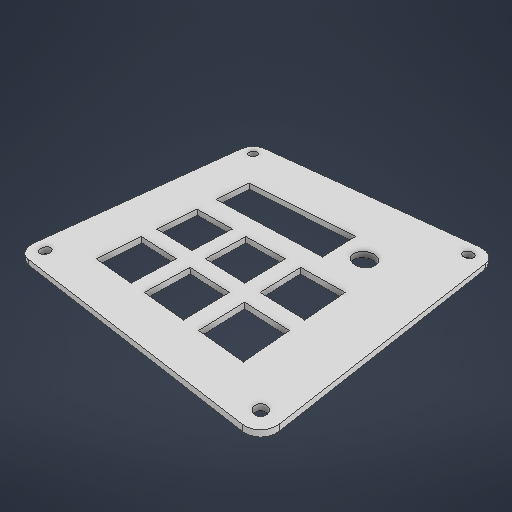
# Autodesk Inventor part: Case_Top
Saved by Autodesk Inventor 2026.1 (Build 301233000, 233)
## iProperties
Created: 2025-12-06
Part Number: Case_Top
Material: Generic
Document SubType Name: Modeling
Designer: chest
Density: 1 g/cm^3
Appearance: Default
Author: chest
Autodesk Inventor part; units mm, degrees
ref_plane "YZ Plane" through (0, 0, 0) normal (1, 0, 0) x (0, 1, 0)
ref_plane "XZ Plane" through (0, 0, 0) normal (0, 1, 0) x (-1, 0, 0)
ref_plane "XY Plane" through (0, 0, 0) normal (0, 0, 1) x (1, 0, 0)
sketch "Sketch1" plane through (0, 0, 0) normal (0, 1, 0) x (-1, 0, 0)
  line L0 (10.136, 16.6006) -> (-75.904, 16.6006)
  line L1 (-75.904, 16.6006) -> (-75.904, -66.8994)
  line L2 (-75.904, -66.8994) -> (10.136, -66.8994)
  line L3 (10.136, -66.8994) -> (10.136, 16.6006)
  point P0 (0, 0)
  dimension "d0" = 86.04
  dimension "d1" = 83.5
  constraints: 8 end point, 2 parallel, 1 horizontal, 1 perpendicular
  measures "d0" distance of L2.end L1.end
  measures "d1" distance of L1.end L0.end
extrude "Extrusion1" add sketch "Sketch1" along normal blind 2
sketch "Sketch2" plane through (0, 2, 0) normal (0, 1, 0) x (1, 0, 0)
  circle A0 centre (-5.136, -11.6006) radius 1.7
  line L0 (-10.136, 66.8994) -> (-10.136, -16.6006) projected
  line L1 (-10.136, -16.6006) -> (75.904, -16.6006) projected
  circle A1 centre (70.904, -11.6006) radius 1.7
  line L2 (75.904, -16.6006) -> (75.904, 66.8994) projected
  circle A2 centre (70.904, 61.8994) radius 1.7
  line L3 (75.904, 66.8994) -> (-10.136, 66.8994) projected
  circle A3 centre (-5.136, 61.8994) radius 1.7
  point P0 (0, 0)
  dimension "d4" = 3.4
  dimension "d5" = 5
  dimension "d6" = 5
  dimension "d7" = 3.4
  dimension "d8" = 5
  dimension "d9" = 5
  dimension "d10" = 3.4
  dimension "d11" = 5
  dimension "d12" = 5
  dimension "d13" = 3.4
  dimension "d14" = 5
  dimension "d15" = 5
  constraints: 4 centre point
  measures "d4" diameter of A0
  measures "d5" distance from line of L0 A0.centre
  measures "d6" distance from line of L1 A0.centre
  measures "d7" diameter of A1
  measures "d8" distance from line of L1 A1.centre
  measures "d9" distance from line of L2 A1.centre
  measures "d10" diameter of A2
  measures "d11" distance from line of L2 A2.centre
  measures "d12" distance from line of L3 A2.centre
  measures "d13" diameter of A3
  measures "d14" distance from line of L3 A3.centre
  measures "d15" distance from line of L0 A3.centre
extrude "Extrusion2" cut sketch "Sketch2" against normal blind 2 contours A0 | A1 | A2 | A3
sketch "Sketch3" plane through (0, 2, 0) normal (0, 1, 0) x (1, 0, 0)
  line L0 (6.834, -4.6006) -> (20.834, -4.6006)
  line L1 (20.834, -4.6006) -> (20.834, 9.3994)
  line L2 (20.834, 9.3994) -> (6.834, 9.3994)
  line L3 (6.834, 9.3994) -> (6.834, -4.6006)
  line L4 (25.884, 9.3994) -> (39.884, 9.3994)
  line L5 (39.884, 9.3994) -> (39.884, -4.6006)
  line L6 (39.884, -4.6006) -> (25.884, -4.6006)
  line L7 (25.884, -4.6006) -> (25.884, 9.3994)
  line L8 (44.934, 9.3994) -> (58.934, 9.3994)
  line L9 (58.934, 9.3994) -> (58.934, -4.6006)
  line L10 (58.934, -4.6006) -> (44.934, -4.6006)
  line L11 (44.934, -4.6006) -> (44.934, 9.3994)
  line L12 (6.834, 14.4494) -> (20.834, 14.4494)
  line L13 (20.834, 14.4494) -> (20.834, 28.4494)
  line L14 (20.834, 28.4494) -> (6.834, 28.4494)
  line L15 (6.834, 28.4494) -> (6.834, 14.4494)
  line L16 (25.884, 28.4494) -> (39.884, 28.4494)
  line L17 (39.884, 28.4494) -> (39.884, 14.4494)
  line L18 (39.884, 14.4494) -> (25.884, 14.4494)
  line L19 (25.884, 14.4494) -> (25.884, 28.4494)
  line L20 (44.934, 28.4494) -> (58.934, 28.4494)
  line L21 (58.934, 28.4494) -> (58.934, 14.4494)
  line L22 (58.934, 14.4494) -> (44.934, 14.4494)
  line L23 (44.934, 14.4494) -> (44.934, 28.4494)
  line L24 (-10.136, 66.8994) -> (-10.136, -16.6006) projected
  line L25 (-10.136, -16.6006) -> (75.904, -16.6006) projected
  line L26 (6.834, 35.5494) -> (45.834, 35.5494)
  line L27 (45.834, 35.5494) -> (45.834, 48.5494)
  line L28 (45.834, 48.5494) -> (6.834, 48.5494)
  line L29 (6.834, 48.5494) -> (6.834, 35.5494)
  circle A0 centre (53.834, 42.0494) radius 3.5
  point P0 (0, 0)
  point P1 (25.884, 21.4494)
  point P2 (20.834, 21.4494)
  point P3 (6.834, 21.4494)
  point P4 (32.884, 9.3994)
  point P5 (32.884, 14.4494)
  point P6 (32.884, -16.6006)
  point P7 (51.934, -4.6006)
  point P8 (13.834, 28.4494)
  point P9 (45.834, 42.0494)
  dimension "d18" = 14
  dimension "d19" = 14
  dimension "d20" = 14
  dimension "d21" = 5.05
  dimension "d22" = 14
  dimension "d23" = 5.05
  dimension "d24" = 14
  dimension "d25" = 14
  dimension "d26" = 5.05
  dimension "d27" = 14
  dimension "d28" = 14
  dimension "d29" = 14
  dimension "d30" = 14
  dimension "d31" = 5.05
  dimension "d32" = 5.05
  dimension "d33" = 5.05
  dimension "d34" = 16.97
  dimension "d35" = 5.05
  dimension "d39" = 12
  dimension "d40" = 12
  dimension "d41" = 12
  dimension "d42" = 39
  dimension "d43" = 13
  dimension "d44" = 7.1
  dimension "d45" = 7
  dimension "d46" = 8
  constraints: 56 end point, 14 parallel, 9 midpoint, 7 horizontal, 7 perpendicular, 1 centre point, 1 point on line
  measures "d18" distance of L2.end L1.end
  measures "d19" distance of L1.end L0.end
  measures "d20" distance of L5.end L6.end
  measures "d21" distance between parallel lines of L1 L7
  measures "d22" distance of L9.end L10.end
  measures "d23" distance between parallel lines of L11 L5
  measures "d24" distance of L14.end L13.end
  measures "d25" distance of L13.end L12.end
  measures "d26" distance between parallel lines of L12 L2
  measures "d27" distance of L17.end L18.end
  measures "d28" distance of L16.end L17.end
  measures "d29" distance of L21.end L22.end
  measures "d30" distance of L20.end L21.end
  measures "d31" distance of point (25.884, 21.449) point (20.834, 21.449)
  measures "d32" distance between parallel lines of L23 L17
  measures "d33" distance between parallel lines of L8 L22
  measures "d34" distance from line of L24 point (6.834, 21.449)
  measures "d35" distance of point (32.884, 9.399) point (32.884, 14.449)
  measures "d39" distance between parallel lines of L0 L25
  measures "d40" distance from line of point (32.884, -16.601) L6
  measures "d41" distance from line of L25 point (51.934, -4.601)
  measures "d42" distance of L28.end L27.end
  measures "d43" distance of L27.end L26.end
  measures "d44" distance from line of point (13.834, 28.449) L26
  measures "d45" diameter of A0
  measures "d46" distance of A0.centre point (45.834, 42.049)
extrude "Extrusion3" cut sketch "Sketch3" against normal blind 2
fillet "Fillet1" radius 5 4 edges at (-10.136, 1, 16.6006) (75.904, 1, 16.6006) (75.904, 1, -66.8994) (-10.136, 1, -66.8994)
body "Solid1"
